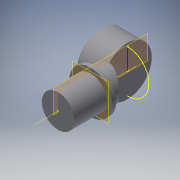
# Autodesk Inventor part: Adjustable elbow piece 1 inch
Saved by Autodesk Inventor 2018 (Build 220112000, 112)
## iProperties
Created: 2018-01-10
Part Number: Adjustable elbow piece 1 inch
Material: Generic
Document SubType Name: Modeling
Designer: owner
Density: 1 g/cm^3
Appearance: Default
Author: owner
Autodesk Inventor part; units mm, degrees
ref_plane "YZ Plane" through (0, 0, 0) normal (1, 0, 0) x (0, 1, 0)
ref_plane "XZ Plane" through (0, 0, 0) normal (0, 1, 0) x (-1, 0, 0)
ref_plane "XY Plane" through (0, 0, 0) normal (0, 0, 1) x (1, 0, 0)
sketch "Sketch1" plane through (0, 0, 0) normal (0, 0, 1) x (1, 0, 0)
  circle A0 centre (0, 0) radius 12.7
  circle A1 centre (0, 0) radius 16.7005
  dimension "d0" = 25.4
  dimension "d1" = 33.401
  constraints: 2 centre point, 2 coincident
  measures "d0" diameter of A0
  measures "d1" diameter of A1
extrude "Extrusion1" add sketch "Sketch1" against normal blind 53.975 contours A0
ref_plane "Work Plane1" through (0, 0, -25.4) normal (0, 0, 1) x (1, 0, 0)
sketch "Sketch3" plane through (0, 0, -25.4) normal (0, 0, 1) x (1, 0, 0)
  circle A0 centre (0, 0) radius 16.7005
  dimension "d6" = 33.401
  constraints: 1 centre point, 1 coincident
  measures "d6" diameter of A0
extrude "Extrusion2" add sketch "Sketch3" against normal blind 3.175
sketch "Sketch4" plane through (0, 0, -53.975) normal (0, 0, -1) x (-1, 0, 0)
  line L0 (0, 0) -> (0, 16.7005)
  circle A0 centre (0, 0) radius 16.7005 projected
  constraints: 2 end point, 1 vertical, 1 vertical alignment, 1 other
ref_plane "Work Plane2" through (0, 0, 0) normal (1, 0, 0) x (0, 0, -1)
sketch "Sketch5" plane through (0, 0, 0) normal (1, 0, 0) x (0, 0, -1)
  line L0 (53.975, -12.7) -> (53.975, 12.7) projected
  circle A0 centre (53.975, 0) radius 19.05
  point P0 (0, 0)
  dimension "d9" = 38.1
  constraints: 1 centre point, 1 midpoint
  measures "d9" diameter of A0
extrude "Extrusion3" cut sketch "Sketch5" along normal blind 12.7
extrude "Extrusion4" add sketch "Sketch5" against normal blind 20.32
body "Solid1"
